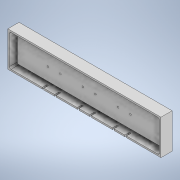
# Autodesk Inventor part: sdm_finger_eit_chamber_mould
Saved by Autodesk Inventor 2021 (Build 250183000, 183)
## iProperties
Created: 2021-05-26
Part Number: sdm_finger_eit_chamber_mould
Material: Generic
Document SubType Name: Modeling
Designer: Charlie
Density: 1 g/cm^3
Appearance: Default
Author: Charlie
Autodesk Inventor part; units mm, degrees
ref_plane "YZ Plane" through (0, 0, 0) normal (1, 0, 0) x (0, 1, 0)
ref_plane "XZ Plane" through (0, 0, 0) normal (0, 1, 0) x (-1, 0, 0)
ref_plane "XY Plane" through (0, 0, 0) normal (0, 0, 1) x (1, 0, 0)
sketch "Sketch2" plane through (0, 0, 0) normal (0, 0, 1) x (1, 0, 0)
  line L0 (-46, 10) -> (46, 10)
  line L1 (47, 9) -> (47, -9)
  line L2 (46, -10) -> (-46, -10)
  line L3 (-47, -9) -> (-47, 9)
  line L4 (-47, 10) -> (47, -10) construction
  line L5 (47, 10) -> (-47, -10) construction
  line L6 (45, 8) -> (-45, 8)
  line L7 (-45, 8) -> (-45, -8)
  line L8 (-45, -8) -> (45, -8)
  line L9 (45, -8) -> (45, 8)
  line L10 (48, 11) -> (-48, 11)
  line L11 (-48, 11) -> (-48, -11)
  line L12 (-48, -11) -> (48, -11)
  line L13 (48, -11) -> (48, 11)
  arc A0 (47, 9) -> (46, 10) centre (46, 9) ccw
  arc A1 (46, -10) -> (47, -9) centre (46, -9) ccw
  arc A2 (-47, -9) -> (-46, -10) centre (-46, -9) ccw
  arc A3 (-46, 10) -> (-47, 9) centre (-46, 9) ccw
  point P0 (0, 0)
  dimension "d0" = 94
  dimension "d1" = 20
  dimension "d2" = 2
  dimension "d3" = 1
  dimension "d10" = 1
  dimension "d40" = 90
  constraints: 28 end point, 8 point on circle, 8 point on line, 8 tangent, 6 parallel, 4 centre point, 3 equal radius, 3 perpendicular, 2 midpoint, 1 horizontal, 6 other
  measures "d0" distance of L4.end L5.end
  measures "d1" distance of L5.start L4.end
  measures "d2" distance between parallel lines of L0 L6
  measures "d3" distance between parallel lines of L0 L10
  measures "d10" radius of A0
  measures "d40" distance of L6.start L6.end
extrude "Extrusion1" add sketch "Sketch2" along normal blind 1 contours L0 A0 L1 A1 L2 A2 L3 A3 | L9 L8 L7 L6 | L13 L12 L11 L10
extrude "Extrusion2" add sketch "Sketch2" along normal blind 7 contours L13 L12 L11 L10
extrude "Extrusion3" add sketch "Sketch2" along normal blind 4 contours L9 L8 L7 L6
sketch "Sketch4" plane through (-48, -11, 0) normal (0, -1, 0) x (1, 0, 0)
  circle A0 centre (22.1132, 6) radius 0.5
  circle A1 centre (29.8868, 6) radius 0.5
  circle A2 centre (44.1132, 6) radius 0.5
  circle A3 centre (51.8842, 6) radius 0.5
  circle A4 centre (66.1132, 6) radius 0.5
  circle A5 centre (73.8868, 6) radius 0.5
  line L0 (0, 6) -> (96, 6)
  line L1 (96, 7) -> (0, 7) projected
  line L2 (22.1132, 4) -> (22.1132, 4)
  line L3 (22.6132, 4.5) -> (22.6132, 8)
  line L4 (22.6132, 8) -> (21.6132, 8)
  line L5 (21.6132, 8) -> (21.6132, 4.5)
  line L6 (21.6132, 4) -> (22.6132, 8) construction
  line L7 (22.6132, 4) -> (21.6132, 8) construction
  line L8 (29.8868, 4) -> (29.8868, 4)
  line L9 (30.3868, 4.5) -> (30.3868, 8)
  line L10 (30.3868, 8) -> (29.3868, 8)
  line L11 (29.3868, 8) -> (29.3868, 4.5)
  line L12 (29.3868, 4) -> (30.3868, 8) construction
  line L13 (30.3868, 4) -> (29.3868, 8) construction
  line L14 (44.1132, 4) -> (44.1132, 4)
  line L15 (44.6132, 4.5) -> (44.6132, 8)
  line L16 (44.6132, 8) -> (43.6132, 8)
  line L17 (43.6132, 8) -> (43.6132, 4.5)
  line L18 (43.6132, 4) -> (44.6132, 8) construction
  line L19 (44.6132, 4) -> (43.6132, 8) construction
  line L20 (51.8842, 4) -> (51.8842, 4)
  line L21 (52.3842, 4.5) -> (52.3842, 8)
  line L22 (52.3842, 8) -> (51.3842, 8)
  line L23 (51.3842, 8) -> (51.3842, 4.5)
  line L24 (51.3842, 4) -> (52.3842, 8) construction
  line L25 (52.3842, 4) -> (51.3842, 8) construction
  line L26 (66.1132, 4) -> (66.1132, 4)
  line L27 (65.6132, 4.5) -> (65.6132, 8)
  line L28 (65.6132, 8) -> (66.6132, 8)
  line L29 (66.6132, 8) -> (66.6132, 4.5)
  line L30 (66.6132, 4) -> (65.6132, 8) construction
  line L31 (65.6132, 4) -> (66.6132, 8) construction
  line L32 (73.8868, 4) -> (73.8868, 4)
  line L33 (73.3868, 4.5) -> (73.3868, 8)
  line L34 (73.3868, 8) -> (74.3868, 8)
  line L35 (74.3868, 8) -> (74.3868, 4.5)
  line L36 (74.3868, 4) -> (73.3868, 8) construction
  line L37 (73.3868, 4) -> (74.3868, 8) construction
  arc A6 (21.6132, 4.5) -> (22.1132, 4) centre (22.1132, 4.5) ccw
  arc A7 (22.1132, 4) -> (22.6132, 4.5) centre (22.1132, 4.5) ccw
  arc A8 (29.3868, 4.5) -> (29.8868, 4) centre (29.8868, 4.5) ccw
  arc A9 (29.8868, 4) -> (30.3868, 4.5) centre (29.8868, 4.5) ccw
  arc A10 (43.6132, 4.5) -> (44.1132, 4) centre (44.1132, 4.5) ccw
  arc A11 (44.1132, 4) -> (44.6132, 4.5) centre (44.1132, 4.5) ccw
  arc A12 (51.3842, 4.5) -> (51.8842, 4) centre (51.8842, 4.5) ccw
  arc A13 (51.8842, 4) -> (52.3842, 4.5) centre (51.8842, 4.5) ccw
  arc A14 (65.6132, 4.5) -> (66.1132, 4) centre (66.1132, 4.5) ccw
  arc A15 (66.1132, 4) -> (66.6132, 4.5) centre (66.1132, 4.5) ccw
  arc A16 (73.3868, 4.5) -> (73.8868, 4) centre (73.8868, 4.5) ccw
  arc A17 (73.8868, 4) -> (74.3868, 4.5) centre (73.8868, 4.5) ccw
  point P0 (96, 0)
  point P1 (69, 6)
  point P2 (71, 6)
  point P3 (49, 6)
  point P4 (47, 6)
  point P5 (27, 6)
  point P6 (25, 6)
  point P7 (22.1132, 4)
  dimension "d59" = 1
  dimension "d60" = 1
  dimension "d61" = 1
  dimension "d62" = 1
  dimension "d63" = 1
  dimension "d64" = 1
  dimension "d65" = 1
  dimension "d66" = 4
  dimension "d67" = 1
  dimension "d68" = 4
  dimension "d69" = 1
  dimension "d70" = 4
  dimension "d71" = 1
  dimension "d72" = 4
  dimension "d73" = 1
  dimension "d74" = 4
  dimension "d75" = 1
  dimension "d76" = 4
  dimension "d81" = 0.5
  constraints: 74 end point, 24 point on circle, 24 point on line, 24 tangent, 18 centre point, 12 midpoint, 12 parallel, 11 equal radius, 6 horizontal, 6 perpendicular
  measures "d59" diameter of A0
  measures "d60" diameter of A1
  measures "d61" diameter of A2
  measures "d62" diameter of A3
  measures "d63" diameter of A4
  measures "d64" diameter of A5
  measures "d65" distance of L4.end L3.end
  measures "d66" distance of L3.end L7.start
  measures "d67" distance of L10.end L9.end
  measures "d68" distance of L9.end L13.start
  measures "d69" distance of L16.end L15.end
  measures "d70" distance of L15.end L19.start
  measures "d71" distance of L22.end L21.end
  measures "d72" distance of L21.end L25.start
  measures "d73" distance of L27.end L28.end
  measures "d74" distance of L31.start L27.end
  measures "d75" distance of L33.end L34.end
  measures "d76" distance of L37.start L33.end
  measures "d81" radius of A6
sketch "Sketch3" plane through (0, 0, 4) normal (0, 0, 1) x (1, 0, 0)
  line L0 (-53.1158, -1) -> (46.8842, -1) construction
  line L1 (43, 0) -> (23, 0) construction
  line L2 (23, 0) -> (23, 5) construction
  line L3 (23, 5) -> (43, 5) construction
  line L4 (43, 5) -> (43, 0) construction
  line L5 (23, 0) -> (23, 5.2137) construction
  line L6 (43, 0) -> (40.1132, 5) construction
  line L7 (46.8842, -1) -> (46.8842, 4.7735) construction
  line L8 (23, 0) -> (25.8868, 5) construction
  line L9 (23, 0) -> (23, 4.6279) construction
  line L10 (21, 0) -> (18.1132, 5) construction
  line L11 (1, 5) -> (21, 5) construction
  line L12 (1, 0) -> (3.8868, 5) construction
  line L13 (-1, 0) -> (-3.8868, 5) construction
  line L14 (-21, 5) -> (-1, 5) construction
  line L15 (-21, 0) -> (-18.1132, 5) construction
  line L16 (-23, 0) -> (-25.8868, 5) construction
  line L17 (-43, 5) -> (-23, 5) construction
  line L18 (-43, 0) -> (-40.1132, 5) construction
  line L19 (43, 5) -> (-43, 5) construction
  line L20 (0, 5) -> (0, 5) construction
  circle A0 centre (-25.8868, 0) radius 0.5
  circle A1 centre (-18.1132, 0) radius 0.5
  circle A2 centre (-3.8868, 0) radius 0.5
  circle A3 centre (3.8842, 0) radius 0.5
  circle A4 centre (18.1132, 0) radius 0.5
  circle A5 centre (25.8868, 0) radius 0.5
  line L21 (-45, 8) -> (-45, -8) projected
  line L22 (45, -8) -> (45, 8) projected
  line L23 (-48, 11) -> (-48, -11) projected
  line L24 (-48, 0) -> (48, 0)
  line L25 (48, -11) -> (48, 11) projected
  point P0 (3.8842, 4)
  dimension "d45" = 20
  dimension "d46" = 5
  dimension "d47" = 30
  dimension "d48" = 30
  dimension "d49" = 22
  dimension "d52" = 0
  dimension "d53" = 1
  dimension "d54" = 1
  dimension "d55" = 1
  dimension "d56" = 1
  dimension "d57" = 1
  dimension "d58" = 1
  constraints: 44 end point, 9 point on line, 6 centre point, 2 midpoint, 2 parallel, 1 collinear, 1 equal length, 1 horizontal, 1 perpendicular, 1 vertical
  measures "d45" distance of L4.end L2.start
  measures "d46" distance of L2.start L2.end
  measures "d47" angle of L7 L6
  measures "d48" angle of L8 L9
  measures "d49" distance of L4.end L10.start
  measures "d52" distance of L20.start L20.end
  measures "d53" diameter of A0
  measures "d54" diameter of A1
  measures "d55" diameter of A2
  measures "d56" diameter of A3
  measures "d57" diameter of A4
  measures "d58" diameter of A5
extrude "Extrusion4" cut sketch "Sketch4" against normal blind 10 contours L0 A0 | L3 A7 A6 L5 A0 | A0 L0 | A0 L5 L1 L3 | L11 L1 L9 A1 | L0 A1 | A1 L0 | A1 L9 A9 A8 L11 | L1 L5 L4 L3 | L11 L10 L9 L1 | L17 L1 L15 A2 | L0 A2 | A2 L0 | A2 L15 A11 A10 L17 | L17 L16 L15 L1 | L23 L1 L21 A3 | L0 A3 | A3 L0 | A3 L21 A13 A12 L23 | L23 L22 L21 L1 | L27 L1 L29 A4 | L0 A4 | A4 L0 | A4 L29 A15 A14 L27 | L27 L28 L29 L1 | L33 L1 L35 A5 | L0 A5 | A5 L0 | A5 L35 A17 A16 L33 | L33 L34 L35 L1
extrude "Extrusion5" cut sketch "Sketch3" against normal blind 10
body "Solid1"
